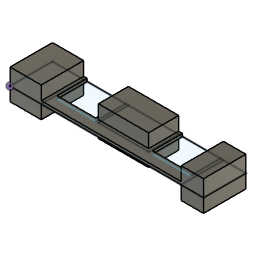
Curtain Connector (Autodesk Fusion 360 design; units mm, degrees)
Autodesk Fusion 360 part; units mm, degrees
sketch "Sketch1" plane through (0, 0, 0) normal (0, 0, 1) x (1, 0, 0)
  line L0 (0, 0) -> (70.8, 0)
  line L1 (70.8, 0) -> (70.8, 15.5)
  line L2 (70.8, 15.5) -> (0, 15.5)
  line L3 (0, 15.5) -> (0, 0)
  line L4 (11.4, 15.5) -> (11.4, 0)
  line L5 (62.6, 15.5) -> (62.6, 0)
  line L6 (27.8, 15.5) -> (27.8, 4.5)
  line L7 (46.2, 15.5) -> (46.2, 4.5)
  line L8 (27.8, 4.5) -> (46.2, 4.5)
  line L9 (12.7, 15.5) -> (12.7, 4.5)
  line L10 (26.8, 15.5) -> (26.8, 4.5)
  line L11 (26.8, 4.5) -> (12.7, 4.5)
  line L12 (47.6, 15.5) -> (47.6, 4.5)
  line L13 (61.5, 15.5) -> (61.5, 4.5)
  line L14 (47.6, 4.5) -> (61.5, 4.5)
  dimension "d1" = 15.5
  dimension "d2" = 70.8
  dimension "d3" = 11.4
  dimension "d4" = 8.2
  dimension "d5" = 43
  dimension "d6" = 46.2
  dimension "d7" = 11
  dimension "d12" = 23.2
  dimension "d13" = 61.5
  dimension "d14" = 26.8
  dimension "d15" = 58.1
  constraint horizontal L0
  constraint vertical L1
  constraint horizontal L2
  constraint vertical L3
  constraint coincident L0.start L3.end
  constraint coincident L2 L4.start
  constraint coincident L0 L4.end
  constraint perpendicular L0 L4
  constraint coincident L2 L5.start
  constraint coincident L0 L5.end
  constraint perpendicular L0 L5
  constraint coincident L2 L6.start
  constraint perpendicular L0 L6
  constraint coincident L2 L7.start
  constraint perpendicular L0 L7
  constraint perpendicular L7 L8
  constraint coincident L2 L9.start
  constraint perpendicular L0 L9
  constraint coincident L2 L10.start
  constraint perpendicular L0 L10
  constraint perpendicular L9 L11
  constraint coincident L2 L12.start
  constraint perpendicular L0 L12
  constraint coincident L2 L13.start
  constraint perpendicular L0 L13
  constraint perpendicular L13 L14
  measures "d1" distance of L0.start L2.end
  measures "d2" distance of L1.end L2.end
  measures "d3" distance of L3 L4
  measures "d4" distance of L1 L5
  measures "d5" distance of L1 L6
  measures "d6" distance of L3 L7
  measures "d7" distance of L2 L8
  measures "d12" distance of L1 L12
  measures "d13" distance of L3 L13
  measures "d14" distance of L3 L10
  measures "d15" distance of L1 L9
extrude "Extrude1" add sketch "Sketch1" along normal blind 1
extrude "Extrude2" add sketch "Sketch1" along normal blind 6 contours L0 L2 L3 L4 | L0 L1 L2 L5 | L2 L6 L7 L8
extrude "Extrude3" cut sketch "Sketch1" along normal blind 1 contours L2 L9 L10 L11 | L2 L12 L13 L14
extrude "Extrude4" add sketch "Sketch1" against normal blind 5 contours L0 L2 L3 L4 | L0 L1 L2 L5 | L2 L6 L7 L8
